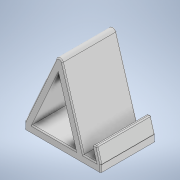
# Autodesk Inventor part: Phone Holder Rev B
Saved by Autodesk Inventor 2021 (Build 250183000, 183)
## iProperties
Created: 2020-09-28
Part Number: Phone Holder Rev B
Material: Generic
Document SubType Name: Modeling
Designer: cmzgt
Density: 1 g/cm^3
Appearance: Default
Author: cmzgt
## iProperties of the stored document _3DPrint.ipt
Created: 2020-09-28
Part Number: _3DPrint
Material: Generic
Document SubType Name: Modeling
Designer: cmzgt
Density: 1 g/cm^3
Appearance: Default
Author: cmzgt
Autodesk Inventor part; units mm, degrees
ref_plane "YZ Plane" through (0, 0, 0) normal (1, 0, 0) x (0, 1, 0)
ref_plane "XZ Plane" through (0, 0, 0) normal (0, 1, 0) x (-1, 0, 0)
ref_plane "XY Plane" through (0, 0, 0) normal (0, 0, 1) x (1, 0, 0)
sketch "Sketch1" plane through (0, 0, 0) normal (0, 1, 0) x (-1, 0, 0)
  line L0 (-38.1, -25.4) -> (38.1, -25.4)
  line L1 (38.1, -25.4) -> (38.1, 25.4)
  line L2 (38.1, 25.4) -> (-38.1, 25.4)
  line L3 (-38.1, 25.4) -> (-38.1, -25.4)
  line L4 (-38.1, -25.4) -> (38.1, 25.4) construction
  line L5 (38.1, -25.4) -> (-38.1, 25.4) construction
  point P0 (0, 0)
  dimension "d0" = 76.2
  dimension "d1" = 50.8
  constraints: 12 end point, 2 midpoint, 2 parallel, 1 horizontal, 1 perpendicular
  measures "d0" distance of L2.end L1.end
  measures "d1" distance of L1.end L0.end
extrude "Extrusion1" add sketch "Sketch1" along normal blind 6.35
sketch "Sketch2" plane through (38.1, 0, -25.4) normal (0, 0, -1) x (-1, 0, 0)
  line L0 (76.2, 6.35) -> (0, 6.35) projected
  line L1 (0, 6.35) -> (21.59, 6.35)
  line L2 (21.59, 6.35) -> (43.642, 79.2894)
  line L3 (76.2, 0) -> (76.2, 6.35) projected
  line L4 (43.642, 79.2894) -> (76.2, 6.35)
  line L5 (76.2, 6.35) -> (69.85, 6.35)
  line L6 (69.85, 6.35) -> (44.8636, 62.3267)
  line L7 (21.59, 6.35) -> (27.94, 6.35) construction
  line L8 (27.94, 6.35) -> (44.8636, 62.3267)
  line L9 (0, 6.35) -> (76.2, 6.35) projected
  line L10 (10.1092, 9.821) -> (9.0598, 6.35)
  line L11 (9.0598, 6.35) -> (5.2498, 6.35)
  line L12 (5.2498, 6.35) -> (9.0598, 19.7904)
  line L13 (9.0598, 19.7904) -> (12.64, 18.7755)
  line L14 (12.64, 18.7755) -> (9.9878, 9.4194)
  point P0 (38.1, 0)
  point P1 (5.2498, 6.35)
  point P2 (9.0598, 6.35)
  dimension "d4" = 21.59
  dimension "d5" = 76.2
  dimension "d6" = 6.35
  dimension "d7" = 6.35
  dimension "d9" = 11.4808
  dimension "d10" = 3.81
  dimension "d11" = 13.97
  constraints: 24 end point, 6 point on line, 2 parallel, 1 perpendicular
  measures "d4" distance of L0.end L1.end
  measures "d5" distance of L1.end L2.end
  measures "d6" distance of L0.start L5.end
  measures "d7" distance of L1.end L7.end
  measures "d9" horizontal distance of L1.end L10.start
  measures "d10" distance of L10.end L11.end
  measures "d11" distance of L11.end L12.end
extrude "Extrusion2" add sketch "Sketch2" against normal up to surface (50.8 mm away) contours L0 L6 L8 L2 L4 | L0 L12 L13 L14 L10
sketch "Sketch3" plane through (0, 6.35, 0) normal (0, 1, 0) x (1, 0, 0)
  line L0 (32.8502, -25.4) -> (38.1, -25.4) projected
  line L1 (38.1, 25.4) -> (32.8502, 25.4) projected
  line L2 (32.8502, -25.4) -> (38.1, -25.4)
  line L3 (38.1, -25.4) -> (38.1, 25.4)
  line L4 (38.1, 25.4) -> (32.8502, 25.4)
  line L5 (32.8502, 25.4) -> (32.8502, -25.4)
  point P0 (0, 0)
  constraints: 8 end point, 2 parallel, 1 horizontal, 1 perpendicular
extrude "Extrusion3" cut sketch "Sketch3" against normal blind 6.35
fillet "Fillet1" radius 1.016 1 edges at (32.8502, 6.35, 0)
fillet "Fillet2" radius 3.175 1 edges at (-5.542, 79.2894, 0)
fillet "Fillet3" radius 3.175 1 edges at (-38.1, 6.35, 0)
fillet "Fillet4" radius 1.016 10 edges at (-5.9152, 73.3838, -25.4) (-23.4195, 39.2385, -25.4) (-38.0303, 6.3352, -25.4) (-38.1, 2.8368, -25.4) (6.7168, 38.742, -25.4) (-5.9152, 73.3838, 25.4) (6.7168, 38.742, 25.4) (-38.0303, 6.3352, 25.4) (-38.1, 2.8368, 25.4) (-23.4195, 39.2385, 25.4)
fillet "Fillet5" radius 1.016 6 edges at (-10.795, 6.35, -25.4) (15.9793, 6.35, -25.4) (22.7751, 6.35, -25.4) (-10.795, 6.35, 25.4) (15.9793, 6.35, 25.4) (22.7751, 6.35, 25.4)
fillet "Fillet6" radius 1.016 4 edges at (27.2501, 19.283, -25.4) (27.2501, 19.283, 25.4) (29.0402, 19.7904, 0) (25.46, 18.7755, 0)
fillet "Fillet7" radius 1.016 8 edges at (32.8405, 6.3487, 25.4) (31.0645, 12.6494, 25.4) (28.8351, 19.423, 25.1024) (32.8502, 3.1044, 25.4) (32.8405, 6.3487, -25.4) (31.0645, 12.6494, -25.4) (28.8351, 19.423, -25.1024) (32.8502, 3.1044, -25.4)
equation "\"d12\" = d7"
body "Solid1"
